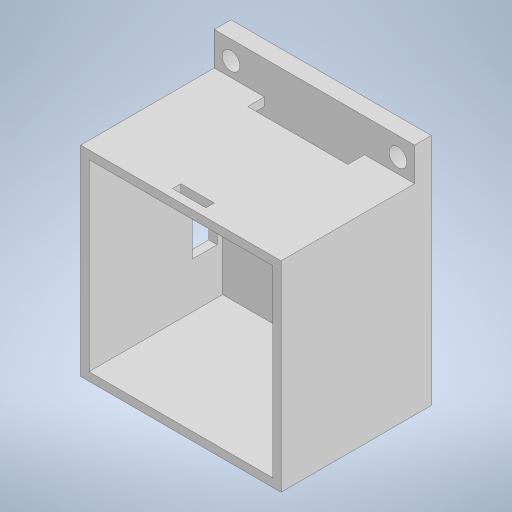
# Autodesk Inventor part: Part_1_box
Saved by Autodesk Inventor 2023 (Build 270158000, 158)
## iProperties
Created: 2023-09-29
Part Number: Part_1_box
Material: Generic
Document SubType Name: Modeling
Designer: zskus
Density: 1 g/cm^3
Appearance: Default
Author: zskus
Autodesk Inventor part; units mm, degrees
ref_plane "YZ Plane" through (0, 0, 0) normal (1, 0, 0) x (0, 1, 0)
ref_plane "XZ Plane" through (0, 0, 0) normal (0, 1, 0) x (-1, 0, 0)
ref_plane "XY Plane" through (0, 0, 0) normal (0, 0, 1) x (1, 0, 0)
sketch "Sketch1" plane through (0, 0, 0) normal (1, 0, 0) x (0, 1, 0)
  line L0 (-38.1, 38.1) -> (38.1, 38.1)
  line L1 (38.1, 38.1) -> (38.1, -38.1)
  line L2 (38.1, -38.1) -> (-38.1, -38.1)
  line L3 (-38.1, -38.1) -> (-38.1, 38.1)
  line L4 (-38.1, 38.1) -> (0, 38.1)
  line L5 (-38.1, 34.925) -> (-38.1, 38.1)
  point P0 (0, 0)
  dimension "d0" = 76.2
  dimension "d1" = 76.2
  dimension "d2" = 38.1
  dimension "d3" = 38.1
  constraints: 12 end point, 2 horizontal, 2 parallel, 1 perpendicular
  measures "d0" distance of L1.end L2.end
  measures "d1" distance of L0.end L1.end
  measures "d2" distance from line of point (0, 0) L0
  measures "d3" distance from line of L1 point (0, 0)
extrude "Extrusion1" add sketch "Sketch1" along normal blind 6.35
sketch "Sketch2" plane through (6.35, 0, 0) normal (1, 0, 0) x (0, 0, -1)
  line L0 (-34.925, 34.925) -> (34.925, 34.925)
  line L1 (34.925, 34.925) -> (34.925, -34.925)
  line L2 (34.925, -34.925) -> (-34.925, -34.925)
  line L3 (-34.925, -34.925) -> (-34.925, 34.925)
  line L4 (38.1, 38.1) -> (-38.1, 38.1) projected
  line L5 (38.1, -38.1) -> (38.1, 38.1) projected
  line L6 (-38.1, 38.1) -> (-38.1, -38.1) projected
  line L7 (-38.1, -38.1) -> (38.1, -38.1) projected
  point P0 (0, 0)
  dimension "d6" = 3.175
  dimension "d7" = 3.175
  dimension "d8" = 3.175
  dimension "d9" = 3.175
  constraints: 8 end point, 2 parallel, 1 horizontal, 1 perpendicular
  measures "d6" distance between parallel lines of L4 L0
  measures "d7" distance between parallel lines of L5 L1
  measures "d8" distance between parallel lines of L6 L3
  measures "d9" distance between parallel lines of L7 L2
extrude "Extrusion2" add sketch "Sketch2" along normal blind 50.8
sketch "Sketch4" plane through (0, -38.1, -38.1) normal (0, 0, -1) x (-1, 0, 0)
  line L0 (0, 0) -> (0, 76.2) projected
  line L1 (0, 76.2) -> (-57.15, 76.2) projected
  line L2 (-57.15, 0) -> (-57.15, 76.2) projected
  line L3 (0, 0) -> (-57.15, 0) projected
  line L4 (-6.35, 3.175) -> (-6.35, 73.025) projected
  line L5 (-8.4284, 41.2742) -> (-17.9534, 41.2742)
  line L6 (-17.9534, 41.2742) -> (-17.9534, 55.5617)
  line L7 (-17.9534, 55.5617) -> (-8.4284, 55.5617)
  line L8 (-8.4284, 55.5617) -> (-8.4284, 41.2742)
  point P0 (0, 38.1)
  dimension "d14" = 14.2875
  dimension "d15" = 9.525
  constraints: 8 end point, 2 parallel, 1 horizontal, 1 perpendicular
  measures "d14" distance of L5.end L6.end
  measures "d15" distance of L5.start L5.end
extrude "Extrusion4" cut sketch "Sketch4" against normal blind 6.35 contours L5 L6 L7 L8
sketch "Sketch5" plane through (0, 0, 0) normal (-1, 0, 0) x (0, 0, 1)
  line L0 (-38.1, 38.1) -> (38.1, 38.1) projected
  line L1 (-38.1, -38.1) -> (-38.1, 38.1) projected
  line L2 (38.1, -38.1) -> (-38.1, -38.1) projected
  line L3 (38.1, 38.1) -> (38.1, -38.1) projected
  line L4 (38.1, -38.1) -> (-38.1, -38.1) projected
  line L5 (38.1, -38.1) -> (-38.1, -38.1)
  line L6 (-38.1, -38.1) -> (-38.1, -50.8)
  line L7 (-38.1, -50.8) -> (38.1, -50.8)
  line L8 (38.1, -50.8) -> (38.1, -38.1)
  circle A0 centre (31.75, -43.6563) radius 3.429
  circle A1 centre (-31.75, -43.6563) radius 3.429
  point P0 (0, 0)
  dimension "d18" = 6.858
  dimension "d19" = 6.858
  dimension "d20" = 63.5
  dimension "d21" = 12.7
  dimension "d22" = 7.1437
  dimension "d23" = 7.1437
  constraints: 8 end point, 2 centre point, 2 parallel, 1 horizontal, 1 perpendicular
  measures "d18" diameter of A0
  measures "d19" diameter of A1
  measures "d20" distance of A1.centre A0.centre
  measures "d21" distance of L5.end L6.end
  measures "d22" distance from line of L7 A1.centre
  measures "d23" distance from line of L7 A0.centre
extrude "Extrusion5" add sketch "Sketch5" against normal blind 6.35 contours L2 L8 L7 L6
sketch "Sketch6" plane through (57.15, -38.1, -38.1) normal (0, -1, 0) x (1, 0, 0)
  line L0 (-50.8, 76.2) -> (-50.8, 0) projected
  line L1 (-50.8, 0) -> (0, 0) projected
  line L2 (0, 76.2) -> (0, 0) projected
  line L3 (-50.8, 76.2) -> (0, 76.2) projected
  line L4 (-57.15, 0) -> (-57.15, 76.2) projected
  line L5 (-57.15, 0) -> (-50.8, 0) projected
  line L6 (-50.8, 76.2) -> (-50.8, 0) projected
  line L7 (-57.15, 76.2) -> (-50.8, 76.2) projected
  line L8 (-50.8, 73.025) -> (-50.8, 3.175) projected
  line L9 (-50.8, 19.05) -> (-44.45, 19.05)
  line L10 (-44.45, 19.05) -> (-44.45, 57.15)
  line L11 (-44.45, 57.15) -> (-50.8, 57.15)
  line L12 (-50.8, 57.15) -> (-50.8, 19.05)
  line L13 (-6.35, 31.75) -> (-3.175, 31.75)
  line L14 (-3.175, 31.75) -> (-3.175, 44.45)
  line L15 (-3.175, 44.45) -> (-6.35, 44.45)
  line L16 (-6.35, 44.45) -> (-6.35, 31.75)
  point P0 (-57.15, 38.1)
  point P1 (-50.8, 38.1)
  point P2 (0, 38.1)
  dimension "d26" = 38.1
  dimension "d27" = 76.2
  dimension "d28" = 38.1
  dimension "d29" = 6.35
  dimension "d32" = 12.7
  dimension "d33" = 3.175
  dimension "d34" = 6.35
  dimension "d35" = 3.175
  constraints: 16 end point, 4 parallel, 2 horizontal, 2 midpoint, 2 perpendicular, 1 point on line
  measures "d26" distance of L9.end L10.end
  measures "d27" distance of L2.start L1.end
  measures "d28" distance from line of L3 point (-50.8, 38.1)
  measures "d29" distance between parallel lines of L0 L10
  measures "d32" distance of L15.end L13.start
  measures "d33" distance of L14.end L15.end
  measures "d34" horizontal distance of point (0, 38.1) L15.end
  measures "d35" distance between parallel lines of L14 L2
extrude "Extrusion6" cut sketch "Sketch6" against normal blind 14.2875 contours L11 L10 L9 L0 | L16 L15 L14 L13
equation "\"d2\" = 0.5 * d1"
equation "\"d3\" = 0.5 * d0"
equation "\"d7\" = d6"
equation "\"d8\" = d6"
equation "\"d9\" = d6"
equation "\"d19\" = d18"
equation "\"d22\" = d23"
equation "\"d28\" = 0.5 * d27"
equation "\"d34\" = 0.5 * d32"
body "Solid1"
